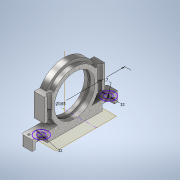
# Autodesk Inventor part: Корпус_Подшипника
Saved by Autodesk Inventor 2021 (Build 250183000, 183)
## iProperties
Created: 2023-04-25
Part Number: Корпус_Подшипника
Material: Сталь, углеродистая
Document SubType Name: Modeling
Designer: gdevc
Density: 7.85 g/cm^3
Appearance: С умеренной полировкой
Mass: 3735.25 g
Surface Area: 918.97 cm^2
Volume: 475.828 cm^3
Author: gdevc
Autodesk Inventor part; units mm, degrees
sketch "Эскиз1" plane through (0, 0, 0) normal (0, 0, 1) x (1, 0, 0)
  line L0 (0, 0) -> (119.1589, 0)
  line L1 (0, 50) -> (52, 50)
  line L2 (52, 50) -> (52, 67.5)
  line L3 (0, 67.5) -> (0, 50)
  line L4 (0, 67.5) -> (15, 67.5)
  line L5 (15, 67.5) -> (15, 60)
  line L6 (15, 60) -> (37, 60)
  line L7 (37, 60) -> (37, 67.5)
  line L8 (37, 67.5) -> (52, 67.5)
  dimension "d0" = 100
  dimension "d1" = 52
  dimension "d2" = 135
  dimension "d3" = 10
  dimension "d4" = 15
  dimension "d5" = 15
  constraints: 18 end point, 5 perpendicular, 3 horizontal, 2 point on line
  measures "d0" diameter of L1 L0
  measures "d1" distance of L1.start L1.end
  measures "d2" diameter of L4 L0
  measures "d3" distance between parallel lines of L1 L6
  measures "d4" distance between parallel lines of L3 L5
  measures "d5" distance between parallel lines of L2 L7
revolve "Вращение1" add sketch "Эскиз1" angle 360 about axis through (0, 0, 0) along (1, 0, 0)
ref_plane "РабПлоскость1" through (0, -67.5, 0) normal (0, 1, 0) x (-1, 0, 0)
sketch "Эскиз3" plane through (0, -67.5, 0) normal (0, 1, 0) x (-1, 0, 0)
  line L0 (0, 0) -> (0, -105)
  line L1 (0, 67.5) -> (0, -67.5) projected
  line L2 (0, -105) -> (-52, -105)
  line L3 (-52, 67.5) -> (-52, -67.5) projected
  line L4 (-52, -105) -> (-52, 47.2217)
  line L5 (0, 105) -> (0, 0)
  line L6 (0, 105) -> (-52, 105)
  line L7 (-52, 105) -> (-52, 44.8764)
  dimension "d15" = 52
  dimension "d16" = 210
  dimension "d17" = 105
  constraints: 12 end point, 1 collinear, 1 horizontal, 1 parallel, 1 perpendicular, 1 point on line
  measures "d15" distance of L0.end L2.end
  measures "d16" distance between parallel lines of L6 L2
  measures "d17" distance from line of L0.start L2
extrude "Выдавливание1" add sketch "Эскиз3" along normal blind 25
sketch "Эскиз2" plane through (0, 0, 0) normal (0, 0, 1) x (1, 0, 0)
  line L0 (9, 50) -> (9, 54)
  line L1 (9, 54) -> (15, 54)
  line L2 (15, 54) -> (15, 50)
  line L3 (42, 50) -> (42, 54)
  line L4 (42, 54) -> (48, 54)
  line L5 (48, 54) -> (48, 50)
  line L6 (52, -67.5) -> (52, 67.5) projected
  line L7 (-10.4, 0) -> (62.4, 0) projected
  line L8 (15, 54) -> (15, 0)
  line L9 (15, -42.5) -> (15, 60) projected
  line L10 (9, 0) -> (9, 50)
  line L11 (48, 50) -> (48, 0)
  line L12 (48, 0) -> (42, 0)
  line L13 (42, 50) -> (42, 0)
  line L14 (52, 50) -> (0, 50) projected
  line L15 (9, 0) -> (15, 0)
  point P0 (0, 0)
  dimension "d7" = 54
  dimension "d8" = 6
  dimension "d9" = 9
  dimension "d10" = 4
  dimension "d11" = 54
  dimension "d12" = 6
  constraints: 24 end point, 5 perpendicular, 5 point on line, 2 vertical, 1 collinear
  measures "d7" distance from line of point (0, 0) L1
  measures "d8" distance between parallel lines of L2 L0
  measures "d9" distance from line of point (0, 0) L0
  measures "d10" distance between parallel lines of L6 L5
  measures "d11" distance from line of point (0, 0) L4
  measures "d12" distance between parallel lines of L5 L3
revolve "Вращение2" cut sketch "Эскиз2" angle 360 about axis through (-10, 0, 0) along (1, 0, 0) contours L14 L8 L7 L10 | L0 L1 L2 L14 | L14 L11 L7 L13 | L3 L4 L5 L14
sketch "Эскиз4" plane through (0, -67.5, -105) normal (-1, 0, 0) x (0, 0, 1)
  arc A0 (131.3391, 25) -> (78.6609, 25) centre (105, 67.5) ccw projected
  arc A1 (157.4404, 25) -> (52.5596, 25) centre (105, 67.5) ccw projected
  circle A2 centre (105, 67.5) radius 50
  point P0 (78.6609, 25)
  constraints: 1 centre point, 1 coincident
extrude "Выдавливание2" cut sketch "Эскиз4" against normal through all
ref_plane "РабПлоскость2" through (0, -42.5, 0) normal (0, 1, 0) x (-1, 0, 0)
sketch "Эскиз5" plane through (0, -42.5, 0) normal (0, 1, 0) x (-1, 0, 0)
  line L0 (-42, -82.5) -> (-10, -82.5) construction
  circle A0 centre (-26, -82.5) radius 8.5
  line L1 (-80.9956, 0) -> (7.5507, 0) construction
  line L2 (-42, 82.5) -> (-10, 82.5) construction
  circle A1 centre (-26, 82.5) radius 8.5
  circle A2 centre (-26, -82.5) radius 16
  circle A3 centre (-26, 82.5) radius 16
  point P0 (0, 0)
  dimension "d23" = 165
  dimension "d28" = 17
  dimension "d79" = 32
  dimension "d80" = 32
  constraints: 6 end point, 4 centre point, 3 symmetric about line, 2 coincident, 1 horizontal, 1 midpoint, 1 other
  measures "d23" diameter of point (0, 0) L0
  measures "d28" diameter of A0
  measures "d79" diameter of A2
  measures "d80" diameter of A3
extrude "Выдавливание4" cut sketch "Эскиз5" against normal through all contours A0 | A1
ref_plane "РабПлоскость3" through (26, -67.5, -105) normal (-1, 0, 0) x (0, 0, 1)
ref_plane "РабПлоскость4" through (0, 18.5, 0) normal (0, 1, 0) x (-1, 0, 0)
extrude "Выдавливание12" cut sketch "Эскиз5" against normal blind 1
sketch "Эскиз14" plane through (0, -67.5, 0) normal (0, -1, 0) x (1, 0, 0)
  line L0 (36, 97.5) -> (16.2132, 97.5)
  line L1 (11, 92.2868) -> (11, 72.5)
  line L2 (16, 67.5) -> (36, 67.5)
  line L3 (41, 72.5) -> (41, 92.5)
  line L4 (80.9956, 0) -> (-7.5507, 0) construction
  circle A0 centre (26, 82.5) radius 8.5 projected
  arc A1 (41, 92.5) -> (36, 97.5) centre (36, 92.5) ccw
  arc A2 (11, 72.5) -> (16, 67.5) centre (16, 72.5) ccw
  arc A3 (36, 67.5) -> (41, 72.5) centre (36, 72.5) ccw
  line L5 (36, -97.5) -> (16, -97.5)
  line L6 (11, -92.5) -> (11, -72.5)
  line L7 (16, -67.5) -> (36, -67.5)
  line L8 (41, -72.5) -> (41, -92.5)
  circle A4 centre (26, -82.5) radius 8.5
  arc A5 (11, -92.5) -> (16, -97.5) centre (16, -92.5) ccw
  arc A6 (16, -67.5) -> (11, -72.5) centre (16, -72.5) ccw
  arc A7 (41, -72.5) -> (36, -67.5) centre (36, -72.5) ccw
  circle A8 centre (11, 97.5) radius 5.2132
  circle A9 centre (26, 82.5) radius 16 projected
  circle A10 centre (41, -97.5) radius 5.2132
  circle A11 centre (26, -82.5) radius 16 projected
  point P0 (0, 0)
  point P1 (11, 67.5)
  point P2 (41, 67.5)
  point P3 (26, 82.5)
  point P4 (11, -67.5)
  point P5 (11, -97.5)
  point P6 (41, -67.5)
  point P7 (26, -82.5)
  point P8 (20.4322, -97.5)
  point P9 (11, -88.0678)
  point P10 (11, -76.9322)
  point P11 (37.3137, -93.8137)
  point P12 (31.5678, -97.5)
  point P13 (35.7868, -97.5)
  point P14 (41, -88.0678)
  point P15 (41, -92.2868)
  point P16 (41, -76.9322)
  dimension "d83" = 30
  dimension "d84" = 30
  dimension "d86" = 5
  dimension "d89" = 15
  constraints: 16 end point, 15 symmetric about line, 14 point on circle, 12 point on line, 9 centre point, 8 tangent, 3 coincident, 2 equal radius, 2 parallel, 1 horizontal, 1 perpendicular, 3 other
  measures "d83" distance of point (11, 97.5) point (11, 67.5)
  measures "d84" distance of point (11, 67.5) point (41, 67.5)
  measures "d86" radius of A1
  measures "d89" horizontal distance of A10.centre A4.centre
extrude "Выдавливание14" cut sketch "Эскиз14" against normal blind 15 contours A1 L3 A9 L0 | A9 L3 L2 L1 L0 | A9 A8 L0 | A9 L1 A8 | L3 A3 L2 A9 | A9 L2 A2 L1 | L5 A11 A10 | L5 A11 L6 L7 L8 | A11 L8 A10 | L5 A5 L6 A11 | A11 L7 A7 L8 | L6 A6 L7 A11
sketch "Эскиз15" plane through (0, -67.5, 0) normal (0, -1, 0) x (1, 0, 0)
  arc A0 (11, 92.2868) -> (16.2132, 97.5) centre (11, 97.5) ccw projected
  arc A1 (41, -92.2868) -> (35.7868, -97.5) centre (41, -97.5) ccw projected
  circle A2 centre (11, 97.5) radius 2.5
  circle A3 centre (41, -97.5) radius 2.5
  point P0 (0, 0)
  dimension "d92" = 5
  dimension "d93" = 5
  constraints: 2 centre point, 2 coincident
  measures "d92" diameter of A2
  measures "d93" diameter of A3
extrude "Выдавливание15" cut sketch "Эскиз15" against normal through all
fillet "Сопряжение3" radius 5 4 edges at (52, -55, 105) (0, -55, 105) (52, -55, -105) (0, -55, -105)
ref_plane "РабПлоскость8" through (0, 32.5, 0) normal (0, -1, 0) x (1, 0, 0)
ref_plane "РабПлоскость9" through (26, 0, 0) normal (1, 0, 0) x (0, 0, -1)
sketch "Эскиз17" plane through (26, 0, 0) normal (1, 0, 0) x (0, 0, -1)
  line L0 (147, 32.5) -> (-147, 32.5) projected
  arc A0 (52.4404, -42.5) -> (-52.4404, -42.5) centre (0, 0) ccw projected
  arc A1 (52.4404, -42.5) -> (-52.4404, -42.5) centre (0, 0) ccw projected
  arc A2 (52.4404, -42.5) -> (-52.4404, -42.5) centre (0, 0) ccw projected
  arc A3 (42.3527, -42.5) -> (-42.3527, -42.5) centre (0, 0) ccw projected
  arc A4 (42.3527, -42.5) -> (-42.3527, -42.5) centre (0, 0) ccw projected
  arc A5 (42.3527, -42.5) -> (-42.3527, -42.5) centre (0, 0) ccw projected
  line L1 (50.4356, 32.5) -> (74, 32.5)
  line L2 (74, 32.5) -> (74, -23.9656)
  line L3 (74, -23.9656) -> (55.0059, -23.9656)
  line L4 (74, -43.5) -> (74, -52.5) projected
  arc A6 (55.0059, -23.9656) -> (50.4356, 32.5) centre (0, 0) ccw
  line L5 (0, 42.0704) -> (0, -31.0307) construction
  line L6 (-50.4356, 32.5) -> (-74, 32.5)
  line L7 (-74, 32.5) -> (-74, -23.9656)
  line L8 (-74, -23.9656) -> (-55.0059, -23.9656)
  arc A7 (-50.4356, 32.5) -> (-55.0059, -23.9656) centre (0, 0) ccw
  point P0 (74, -48)
  point P1 (50.4356, 32.5)
  point P2 (-50.4356, 32.5)
  constraints: 14 end point, 6 point on circle, 6 symmetric about line, 3 point on line, 2 centre point, 2 vertical, 1 coincident, 1 midpoint, 1 perpendicular, 1 other
extrude "Выдавливание16" add sketch "Эскиз17" along normal mid plane 52 contours L0 A0 L3 A3 | A3 L8 A0 L0 | L0 L2 L3 A0 | A0 L8 L7 L0
sketch "Эскиз18" plane through (0, 32.5, 74) normal (0, 1, 0) x (1, 0, 0)
  circle A0 centre (26, -8.5) radius 8.5 projected
  line L0 (0, 0) -> (52, 0) projected
  circle A1 centre (26, 12) radius 6
  circle A2 centre (26, 12) radius 5
  circle A3 centre (26, 136) radius 6
  circle A4 centre (26, 136) radius 5
  line L1 (0, 148) -> (52, 148) projected
  point P0 (0, 74)
  dimension "d100" = 12
  dimension "d101" = 10
  dimension "d102" = 12
  dimension "d103" = 12
  dimension "d104" = 10
  dimension "d105" = 12
  constraints: 4 centre point, 1 coincident
  measures "d100" diameter of A1
  measures "d101" diameter of A2
  measures "d102" distance from line of A1.centre L0
  measures "d103" diameter of A3
  measures "d104" diameter of A4
  measures "d105" distance from line of L1 A3.centre
extrude "Выдавливание17" cut sketch "Эскиз18" against normal blind 62 contours A2 | A4
extrude "Выдавливание18" cut sketch "Эскиз18" against normal blind 35 contours A1 | A3
thread "Резьба5" size "M10x1.5" class "6H" standard "ISO Metric profile" length 25
thread "Резьба6" size "M10x1.5" class "6H" standard "ANSI Metric M Profile" length 25
chamfer "Фаска3" distance 0.5 angle 45 1 edges at (21, -2.5, 62)
chamfer "Фаска4" distance 0.5 angle 45 1 edges at (21, -2.5, -62)
equation "\"d17\" = 0.5 * d16"
